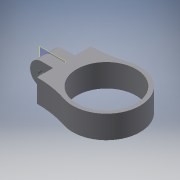
# Autodesk Inventor part: wrenchB
Saved by Autodesk Inventor 2017 (Build 210142000, 142)
## iProperties
Created: 2017-02-16
Part Number: wrenchB
Material: Generic
Document SubType Name: Modeling
Designer: kingb
Density: 1 g/cm^3
Appearance: Chrome - Polished
Author: kingb
Autodesk Inventor part; units mm, degrees
ref_plane "YZ Plane" through (0, 0, 0) normal (1, 0, 0) x (0, 1, 0)
sketch "Sketch2" plane through (0, 0, 0) normal (0, 0, 1) x (1, 0, 0)
  arc A0 (4.191, -4.318) -> (4.191, 4.318) centre (4.191, 0) ccw projected
  arc A1 (4.191, 4.318) -> (4.191, -4.318) centre (4.191, 0) ccw
  circle A2 centre (4.191, 0) radius 1.397 projected
  line L0 (8.509, 0) -> (8.509, 4.318)
  line L1 (8.509, 4.318) -> (4.191, 4.318)
  line L2 (8.509, 0) -> (8.509, -4.318)
  line L3 (8.509, -4.318) -> (4.191, -4.318)
  point P0 (0, 0)
  constraints: 8 end point, 7 tangent, 3 point on circle, 2 perpendicular, 2 point on line, 1 centre point, 1 coincident, 1 vertical
ref_plane "Work Plane1" through (0, -4.064, 8.255) normal (0, 0, -1) x (0, 1, 0)
extrude "Extrusion1" add sketch "Sketch2" along normal up to surface (8.255 mm away)
ref_plane "Work Plane2" through (0, 0, 4.1275) normal (0, 0, -1) x (-1, 0, 0)
sketch "Sketch3" plane through (4.191, -4.318, 0) normal (0, -1, 0) x (1, 0, 0)
  circle A0 centre (20.32, 4.1275) radius 12.7
  line L0 (40.4876, 4.1275) -> (-11.7856, 4.1275) projected
  line L1 (4.318, 0) -> (4.318, 8.255) projected
  circle A1 centre (20.32, 4.1275) radius 11.176
  line L2 (0, 14.2875) -> (4.064, 14.2875) projected
  line L3 (4.064, -6.0325) -> (0, -6.0325) projected
  line L4 (0, 0) -> (4.318, 0) projected
  line L5 (4.318, 0) -> (4.318, -6.0386)
  line L6 (4.318, 8.255) -> (4.318, 14.2875)
  arc A2 (4.318, 14.2875) -> (16.3873, 16.2033) centre (4.318, 53.2638) ccw
  arc A3 (16.3963, -7.9512) -> (4.318, -6.0386) centre (4.318, -45.1333) ccw
  point P0 (-4.191, 0)
  dimension "d2" = 25.4
  dimension "d3" = 0
  dimension "d4" = 16.002
  dimension "d5" = 1.524
  dimension "d8" = 0
  dimension "d9" = 0.0061
  constraints: 6 point on circle, 4 centre point, 4 end point, 2 line through centre, 2 tangent, 2 vertical
  measures "d2" diameter of A0
  measures "d3" distance from line of L0 A1.centre
  measures "d4" distance from line of L1 A1.centre
  measures "d5" radial gap between concentric circles of A0 A1
  measures "d8" vertical distance of L2.end L6.end
  measures "d9" vertical distance of L3.start L5.end
extrude "Extrusion2" add sketch "Sketch3" against normal up to surface (8.636 mm away) contours L0 A1 A0 | A0 L0 A1 | A0 L0 L1 L6 A2 | A3 L5 L1 L0 A0
fillet "Fillet1" radius 0.254 12 edges at (8.509, 4.318, -3.0193) (8.509, 4.318, 11.2712) (8.509, 0, -6.0386) (8.509, -4.318, -3.0193) (8.509, -4.318, 11.2712) (8.509, 0, 14.2875) (37.211, -4.318, 4.1322) (14.6234, -4.318, -6.5197) (14.6192, -4.318, 14.7694) (37.211, 4.318, 4.1322) (14.6234, 4.318, -6.5197) (14.6192, 4.318, 14.7694)
body "Solid1"
